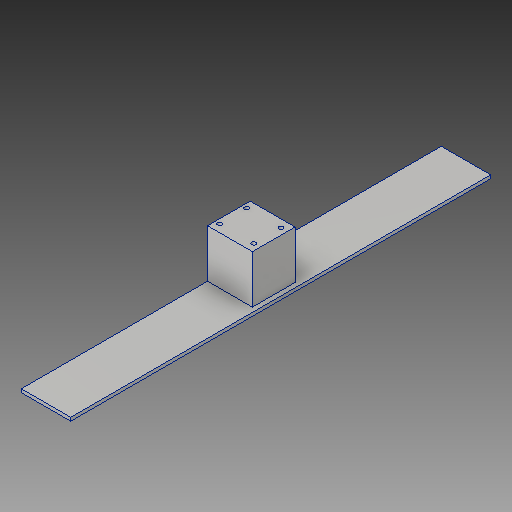
# Autodesk Inventor part: claw mount
Saved by Autodesk Inventor 2017 (Build 210142000, 142)
## iProperties
Created: 2018-02-03
Part Number: claw mount
Material: Aluminum 6061
Document SubType Name: Modeling
Designer: S338674153
Density: 2.7 g/cm^3
Appearance: Aluminum - Flat
Author: S338674153
Autodesk Inventor part; units mm, degrees
ref_plane "YZ Plane" through (0, 0, 0) normal (1, 0, 0) x (0, 1, 0)
ref_plane "XZ Plane" through (0, 0, 0) normal (0, 1, 0) x (-1, 0, 0)
ref_plane "XY Plane" through (0, 0, 0) normal (0, 0, 1) x (1, 0, 0)
sketch "Sketch1" plane through (0, 0, 0) normal (0, 1, 0) x (-1, 0, 0)
  line L0 (0, 0) -> (46.3296, 0)
  line L1 (46.3296, 0) -> (46.3296, -393.7)
  line L2 (46.3296, -393.7) -> (0, -393.7)
  line L3 (0, -393.7) -> (0, 0)
  dimension "d0" = 46.3296
  dimension "d1" = 393.7
  constraints: 8 end point, 2 parallel, 1 horizontal, 1 perpendicular
  measures "d0" distance of L1.end L2.end
  measures "d1" distance of L0.end L1.end
extrude "Extrusion1" add sketch "Sketch1" along normal blind 3.175
sketch "Sketch2" plane through (0, 3.175, 0) normal (0, 1, 0) x (1, 0, 0)
  circle A0 centre (-42.3418, 181.864) radius 2.0193
  line L0 (-46.3296, 0) -> (-46.3296, 393.7) projected
  line L1 (-46.3296, 0) -> (0, 0) projected
  circle A1 centre (-42.3418, 207.264) radius 1.9939
  circle A2 centre (-10.2108, 181.864) radius 1.9939
  circle A3 centre (-10.2108, 207.264) radius 1.9939
  line L2 (-46.3296, 393.7) -> (-46.3296, 0) projected
  line L3 (-42.3418, 181.864) -> (-42.3418, 174.5742)
  line L4 (-46.3296, 174.5742) -> (-4.2672, 174.5742)
  line L5 (-4.2672, 174.5742) -> (-4.2672, 214.5792)
  line L6 (-4.2672, 214.5792) -> (-46.3296, 214.5792)
  line L7 (-46.3296, 174.5742) -> (-46.3296, 214.5792)
  dimension "d4" = 4.0386
  dimension "d5" = 3.9878
  dimension "d6" = 181.864
  dimension "d8" = 3.9878
  dimension "d10" = 3.9878
  dimension "d12" = 3.9878
  dimension "d14" = 7.2898
  dimension "d15" = 42.0624
  dimension "d16" = 40.005
  constraints: 10 end point, 4 centre point, 2 perpendicular, 2 point on line, 2 vertical, 1 collinear
  measures "d4" diameter of A0
  measures "d5" distance from line of L0 L3.start
  measures "d6" distance from line of L1 L3.start
  measures "d8" diameter of A1
  measures "d10" diameter of A2
  measures "d12" diameter of A3
  measures "d14" distance of L3.start L3.end
  measures "d15" distance of L4.start L4.end
  measures "d16" distance of L4.end L5.end
extrude "Extrusion2" add sketch "Sketch2" along normal blind 45.04
body "Solid1"
